Autodesk Fusion 360 part; units mm, degrees
note: some values were not read from the file. Set by a fixed rule: which sketch regions a step uses.
(part 5 of 5)
  line L1562 (-145.873, -75.7002) -> (-146.0412, -75.9619)
  line L1563 (-146.0412, -75.9619) -> (-146.2219, -76.2125)
  line L1564 (-146.2219, -76.2125) -> (-146.4149, -76.4518)
  line L1565 (-146.4149, -76.4518) -> (-146.6201, -76.6795)
  line L1566 (-146.6201, -76.6795) -> (-146.8374, -76.8954)
  line L1567 (-146.8374, -76.8954) -> (-147.0665, -77.0991)
  line L1568 (-147.0665, -77.0991) -> (-147.3075, -77.2905)
  line L1569 (-147.3075, -77.2905) -> (-147.56, -77.4693)
  line L1570 (-147.56, -77.4693) -> (-147.824, -77.6353)
  line L1571 (-147.824, -77.6353) -> (-148.0994, -77.7881)
  line L1572 (-148.0994, -77.7881) -> (-148.386, -77.9276)
  line L1573 (-148.386, -77.9276) -> (-148.6836, -78.0535)
  line L1574 (-148.6836, -78.0535) -> (-148.9921, -78.1655)
  line L1575 (-148.9921, -78.1655) -> (-149.3113, -78.2634)
  line L1576 (-149.3113, -78.2634) -> (-149.6412, -78.3469)
  line L1577 (-149.6412, -78.3469) -> (-149.9816, -78.4158)
  line L1578 (-149.9816, -78.4158) -> (-150.3322, -78.4698)
  line L1579 (-150.3322, -78.4698) -> (-150.6931, -78.5087)
  line L1580 (-150.6931, -78.5087) -> (-151.064, -78.5322)
  line L1581 (-151.064, -78.5322) -> (-151.4448, -78.5402)
  line L1582 (-151.4448, -78.5402) -> (-151.8143, -78.5322)
  line L1583 (-151.8143, -78.5322) -> (-152.1737, -78.5079)
  line L1584 (-152.1737, -78.5079) -> (-152.5229, -78.4681)
  line L1585 (-152.5229, -78.4681) -> (-152.8617, -78.4132)
  line L1586 (-152.8617, -78.4132) -> (-153.19, -78.3438)
  line L1587 (-153.19, -78.3438) -> (-153.5078, -78.2604)
  line L1588 (-153.5078, -78.2604) -> (-153.8149, -78.1635)
  line L1589 (-153.8149, -78.1635) -> (-154.1113, -78.0537)
  line L1590 (-154.1113, -78.0537) -> (-154.3968, -77.9313)
  line L1591 (-154.3968, -77.9313) -> (-154.6713, -77.797)
  line L1592 (-154.6713, -77.797) -> (-154.9347, -77.6512)
  line L1593 (-154.9347, -77.6512) -> (-155.1869, -77.4945)
  line L1594 (-155.1869, -77.4945) -> (-155.4279, -77.3274)
  line L1595 (-155.4279, -77.3274) -> (-155.6574, -77.1504)
  line L1596 (-155.6574, -77.1504) -> (-155.8755, -76.964)
  line L1597 (-155.8755, -76.964) -> (-156.082, -76.7687)
  line L1598 (-156.082, -76.7687) -> (-156.2767, -76.5651)
  line L1599 (-156.2767, -76.5651) -> (-156.4597, -76.3536)
  line L1600 (-156.4597, -76.3536) -> (-156.6307, -76.1348)
  line L1601 (-156.6307, -76.1348) -> (-156.7897, -75.9092)
  line L1602 (-156.7897, -75.9092) -> (-156.9366, -75.6773)
  line L1603 (-156.9366, -75.6773) -> (-157.0712, -75.4395)
  line L1604 (-157.0712, -75.4395) -> (-157.1936, -75.1965)
  line L1605 (-157.1936, -75.1965) -> (-157.3035, -74.9488)
  line L1606 (-157.3035, -74.9488) -> (-157.4009, -74.6967)
  line L1607 (-157.4009, -74.6967) -> (-157.4856, -74.441)
  line L1608 (-157.4856, -74.441) -> (-157.5576, -74.182)
  line L1609 (-157.5576, -74.182) -> (-157.6167, -73.9203)
  line L1610 (-157.6167, -73.9203) -> (-157.6629, -73.6565)
  line L1611 (-157.6629, -73.6565) -> (-157.696, -73.3909)
  line L1612 (-157.696, -73.3909) -> (-157.7159, -73.1242)
  line L1613 (-157.7159, -73.1242) -> (-157.7229, -72.8568)
  line L1614 (-157.7229, -72.8568) -> (-157.7189, -72.6442)
  line L1615 (-157.7189, -72.6442) -> (-157.7056, -72.4512)
  line L1616 (-157.7056, -72.4512) -> (-157.6826, -72.2773)
  line L1617 (-157.6826, -72.2773) -> (-157.6493, -72.1214)
  line L1618 (-157.6493, -72.1214) -> (-157.605, -71.9829)
  line L1619 (-157.605, -71.9829) -> (-157.549, -71.8607)
  line L1620 (-157.549, -71.8607) -> (-157.4807, -71.7542)
  line L1621 (-157.4807, -71.7542) -> (-157.3994, -71.6624)
  line L1622 (-157.3994, -71.6624) -> (-157.3044, -71.5845)
  line L1623 (-157.3044, -71.5845) -> (-157.195, -71.5197)
  line L1624 (-157.195, -71.5197) -> (-157.0707, -71.4672)
  line L1625 (-157.0707, -71.4672) -> (-156.9307, -71.4261)
  line L1626 (-156.9307, -71.4261) -> (-156.7744, -71.3956)
  line L1627 (-156.7744, -71.3956) -> (-156.6012, -71.3747)
  line L1628 (-156.6012, -71.3747) -> (-156.4103, -71.3628)
  line L1629 (-156.4103, -71.3628) -> (-156.201, -71.3588)
  line L1630 (-156.201, -71.3588) -> (-155.9608, -71.3588)
  line L1631 (-155.9608, -71.3588) -> (-155.841, -71.3363)
  line L1632 (-155.841, -71.3363) -> (-155.7174, -71.3283)
  line L1633 (-155.7174, -71.3283) -> (-151.0533, -71.3283)
  line L1634 (-151.0533, -71.3283) -> (-150.9298, -71.3363)
  line L1635 (-150.9298, -71.3363) -> (-150.8102, -71.3588)
  line L1636 (-150.8102, -71.3588) -> (-150.7901, -71.3559)
  line L1637 (-150.7901, -71.3559) -> (-150.7911, -71.3619)
  line L1638 (-150.7911, -71.3619) -> (-150.6265, -71.419)
  arc A0 (-200, -134) -> (-199, -135) centre (-199, -134) ccw
  line L1639 (-199, -135) -> (-151, -135)
  arc A1 (-150, -136) -> (-151, -135) centre (-151, -136) ccw
  line L1640 (-150, -136) -> (-150, -164)
  arc A2 (-150, -164) -> (-149, -165) centre (-149, -164) ccw
  line L1641 (-149, -165) -> (-1, -165)
  arc A3 (-1, -165) -> (0, -164) centre (-1, -164) ccw
  line L1642 (0, -164) -> (0, -1)
  arc A4 (0, -1) -> (-1, 0) centre (-1, -1) ccw
  line L1643 (-1, 0) -> (-199, 0)
  arc A5 (-199, 0) -> (-200, -1) centre (-199, -1) ccw
  line L1644 (-200, -1) -> (-200, -134)
  circle A6 centre (-195, -42) radius 1.5
  circle A7 centre (-195, -111) radius 1.5
  circle A8 centre (-30, -111) radius 1.5
  circle A9 centre (-30, -42) radius 1.5
component "PCB Cover" placed x (1, 0, 0) y (0, 1, 0) z (0, 0, 1) at (0, 0, 0)
equation "Hole = 3 mm"
equation "d8_1 = Hole"
equation "d9_1 = Hole"
equation "d10_1 = Hole"
equation "d11_1 = Hole"
